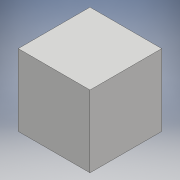
# Autodesk Inventor part: CalibrationCube
Saved by Autodesk Inventor 2017 (Build 210142000, 142)
## iProperties
Created: 2018-12-06
Part Number: CalibrationCube
Material: Generic
Document SubType Name: Modeling
Designer: Eric the Great
Density: 1 g/cm^3
Appearance: Default
Author: Eric the Great
Autodesk Inventor part; units mm, degrees
ref_plane "YZ Plane" through (0, 0, 0) normal (1, 0, 0) x (0, 1, 0)
ref_plane "XZ Plane" through (0, 0, 0) normal (0, 1, 0) x (-1, 0, 0)
ref_plane "XY Plane" through (0, 0, 0) normal (0, 0, 1) x (1, 0, 0)
sketch "Sketch1" plane through (0, 0, 0) normal (0, 1, 0) x (-1, 0, 0)
  line L0 (-28.325, 28.325) -> (28.325, 28.325)
  line L1 (28.325, 28.325) -> (28.325, -28.325)
  line L2 (28.325, -28.325) -> (-28.325, -28.325)
  line L3 (-28.325, -28.325) -> (-28.325, 28.325)
  line L4 (-28.325, 28.325) -> (28.325, -28.325) construction
  line L5 (28.325, 28.325) -> (-28.325, -28.325) construction
  point P0 (0, 0)
  dimension "d1" = 56.65
  constraints: 12 end point, 2 midpoint, 2 parallel, 2 perpendicular, 1 horizontal
  measures "d1" distance of L0.end L1.end
extrude "Extrusion1" add sketch "Sketch1" along normal blind 56.65
sketch "Sketch2" plane through (0, 56.65, 0) normal (0, 1, 0) x (1, 0, 0)
  line L0 (-16.1842, -24.3423) -> (-16.1842, 20.4869) construction
  line L1 (-16.1842, 20.4869) -> (-7.9053, 20.4869) construction
  line L2 (-7.9053, 20.4869) -> (-7.9053, -24.3423) construction
  line L3 (-7.9053, -24.3423) -> (-16.1842, -24.3423) construction
  line L4 (-0.0592, -21.5544) -> (-0.0592, 23.2747) construction
  line L5 (-0.0592, 23.2747) -> (5.9092, 23.2747) construction
  line L6 (5.9092, 23.2747) -> (5.9092, -21.5544) construction
  line L7 (5.9092, -21.5544) -> (-0.0592, -21.5544) construction
  line L8 (-8.6359, -18.0855) -> (-8.6359, -19.371)
  line L9 (-8.6359, -19.371) -> (-11.6211, -21.3753)
  line L10 (-11.6211, -21.3753) -> (-11.6211, -22.3927)
  line L11 (-11.6211, -22.3927) -> (-8.6359, -22.3927)
  line L12 (-8.6359, -22.3927) -> (-8.6359, -23.4345)
  line L13 (-8.6359, -23.4345) -> (-15.6359, -23.4345)
  line L14 (-15.6359, -23.4345) -> (-15.6359, -20.9793)
  spline S0 degree 2 poles (-15.6359, -20.9793) (-15.6359, -19.6634) (-15.1059, -18.5181) (-14.2652, -18.5181) knots 0 0 0 1 2 2 2
  line L15 (-14.2652, -18.5181) -> (-13.0589, -18.5181)
  spline S1 degree 2 poles (-13.0589, -18.5181) (-12.4131, -18.5181) (-11.7552, -19.5781) (-11.7552, -20.3336) knots 0 0 0 1 2 2 2
  line L16 (-11.7552, -20.3336) -> (-8.6359, -18.0855)
  line L17 (-13.1868, -19.5659) -> (-14.1555, -19.5659)
  spline S2 degree 2 poles (-14.1555, -19.5659) (-14.9414, -19.5659) (-14.9414, -20.9245) knots 0 0 0 1 1 1
  line L18 (-14.9414, -20.9245) -> (-14.9414, -22.3927)
  line L19 (-14.9414, -22.3927) -> (-12.3157, -22.3927)
  line L20 (-12.3157, -22.3927) -> (-12.3157, -21.022)
  spline S3 degree 2 poles (-12.3157, -21.022) (-12.3157, -20.2787) (-12.6812, -19.5659) (-13.1868, -19.5659) knots 0 0 0 1 2 2 2
  line L21 (-12.0963, -12.2857) -> (-10.2869, -12.2857)
  spline S4 degree 2 poles (-10.2869, -12.2857) (-9.7996, -12.2857) (-9.1294, -12.5233) (-8.7639, -12.8888) (-8.5689, -13.5712) (-8.5263, -14.1865) (-8.5263, -14.6921) knots 0 0 0 1 2 3 4 5 5 5
  spline S5 degree 2 poles (-8.5263, -14.6921) (-8.5263, -15.3379) (-8.6116, -16.0629) (-8.9466, -16.7818) (-9.6838, -17.0986) (-10.2869, -17.0986) knots 0 0 0 1 2 3 4 4 4
  line L22 (-10.2869, -17.0986) -> (-12.0963, -17.0986)
  spline S6 degree 2 poles (-12.0963, -17.0986) (-12.6142, -17.0986) (-13.327, -16.8488) (-13.7169, -16.4954) (-13.9179, -15.8009) (-13.9606, -15.21) (-13.9606, -14.1743) (-13.9179, -13.5833) (-13.7169, -12.8888) (-13.327, -12.5355) (-12.6142, -12.2857) (-12.0963, -12.2857) knots 0 0 0 1 2 3 4 5 6 7 8 9 10 10 10
  line L23 (-10.1468, -13.2787) -> (-12.2608, -13.2787)
  spline S7 degree 2 poles (-12.2608, -13.2787) (-12.9797, -13.2787) (-13.327, -13.8636) (-13.327, -15.5207) (-12.9797, -16.1055) (-12.2608, -16.1055) knots 0 0 0 1 2 3 4 4 4
  line L24 (-12.2608, -16.1055) -> (-10.1468, -16.1055)
  spline S8 degree 2 poles (-10.1468, -16.1055) (-9.7996, -16.1055) (-9.3914, -15.9532) (-9.2086, -15.5451) (-9.166, -15.1125) (-9.166, -14.2718) (-9.2086, -13.8392) (-9.3914, -13.431) (-9.7996, -13.2787) (-10.1468, -13.2787) knots 0 0 0 1 2 3 4 5 6 7 8 8 8
  line L25 (-12.4862, -6.0229) -> (-10.3418, -6.0229)
  spline S9 degree 2 poles (-10.3418, -6.0229) (-9.8666, -6.0229) (-9.1781, -6.3031) (-8.8004, -6.7235) (-8.5811, -7.418) (-8.5263, -8.0211) (-8.5263, -8.4537) knots 0 0 0 1 2 3 4 5 5 5
  spline S10 degree 2 poles (-8.5263, -8.4537) (-8.5263, -9.0142) (-8.6359, -9.7209) (-8.9832, -10.4337) (-9.7447, -10.7809) (-10.3418, -10.7809) knots 0 0 0 1 2 3 4 4 4
  line L26 (-10.3418, -10.7809) -> (-16.1842, -10.7809)
  line L27 (-16.1842, -10.7809) -> (-16.1842, -9.8122)
  line L28 (-16.1842, -9.8122) -> (-14.6185, -9.8122)
  spline S11 degree 2 poles (-14.6185, -9.8122) (-14.4175, -9.8122) (-13.5828, -9.8183) (-13.3818, -9.8183) knots 0 0 0 1 2 2 2
  spline S12 degree 2 poles (-13.3818, -9.8183) (-13.6316, -9.7757) (-13.9606, -8.9715) (-13.9606, -8.1795) knots 0 0 0 1 2 2 2
  spline S13 degree 2 poles (-13.9606, -8.1795) (-13.9606, -6.0229) (-12.4862, -6.0229) knots 0 0 0 1 1 1
  line L29 (-10.2016, -7.0159) -> (-12.2486, -7.0159)
  spline S14 degree 2 poles (-12.2486, -7.0159) (-12.9188, -7.0159) (-13.2721, -7.6434) (-13.2721, -8.4415) knots 0 0 0 1 2 2 2
  spline S15 degree 2 poles (-13.2721, -8.4415) (-13.2721, -9.2091) (-12.864, -9.8122) (-12.2486, -9.8122) knots 0 0 0 1 2 2 2
  line L30 (-12.2486, -9.8122) -> (-10.2016, -9.8122)
  spline S16 degree 2 poles (-10.2016, -9.8122) (-9.5437, -9.8122) (-9.166, -9.2152) (-9.166, -8.4293) knots 0 0 0 1 2 2 2
  spline S17 degree 2 poles (-9.166, -8.4293) (-9.166, -7.6312) (-9.5437, -7.0159) (-10.2016, -7.0159) knots 0 0 0 1 2 2 2
  line L31 (-12.0963, 0.0816) -> (-10.2869, 0.0816)
  spline S18 degree 2 poles (-10.2869, 0.0816) (-9.7996, 0.0816) (-9.1294, -0.156) (-8.7639, -0.5216) (-8.5689, -1.2039) (-8.5263, -1.8192) (-8.5263, -2.3249) knots 0 0 0 1 2 3 4 5 5 5
  spline S19 degree 2 poles (-8.5263, -2.3249) (-8.5263, -2.9706) (-8.6116, -3.6956) (-8.9466, -4.4145) (-9.6838, -4.7313) (-10.2869, -4.7313) knots 0 0 0 1 2 3 4 4 4
  line L32 (-10.2869, -4.7313) -> (-12.0963, -4.7313)
  spline S20 degree 2 poles (-12.0963, -4.7313) (-12.6142, -4.7313) (-13.327, -4.4815) (-13.7169, -4.1282) (-13.9179, -3.4337) (-13.9606, -2.8427) (-13.9606, -1.807) (-13.9179, -1.2161) (-13.7169, -0.5216) (-13.327, -0.1682) (-12.6142, 0.0816) (-12.0963, 0.0816) knots 0 0 0 1 2 3 4 5 6 7 8 9 10 10 10
  line L33 (-10.1468, -0.9115) -> (-12.2608, -0.9115)
  spline S21 degree 2 poles (-12.2608, -0.9115) (-12.9797, -0.9115) (-13.327, -1.4963) (-13.327, -3.1534) (-12.9797, -3.7383) (-12.2608, -3.7383) knots 0 0 0 1 2 3 4 4 4
  line L34 (-12.2608, -3.7383) -> (-10.1468, -3.7383)
  spline S22 degree 2 poles (-10.1468, -3.7383) (-9.7996, -3.7383) (-9.3914, -3.586) (-9.2086, -3.1778) (-9.166, -2.7452) (-9.166, -1.9045) (-9.2086, -1.4719) (-9.3914, -1.0638) (-9.7996, -0.9115) (-10.1468, -0.9115) knots 0 0 0 1 2 3 4 5 6 7 8 8 8
  spline S23 degree 2 poles (-8.6786, 5.3636) (-8.5263, 4.6508) (-8.5263, 3.6882) knots 0 0 0 1 1 1
  spline S24 degree 2 poles (-8.5263, 3.6882) (-8.5263, 3.213) (-8.5628, 2.6891) (-8.7456, 2.0067) (-9.0868, 1.6534) (-9.7447, 1.3914) (-10.2321, 1.3914) knots 0 0 0 1 2 3 4 5 5 5
  line L35 (-10.2321, 1.3914) -> (-12.1512, 1.3914)
  spline S25 degree 2 poles (-12.1512, 1.3914) (-12.5837, 1.3914) (-13.2051, 1.5559) (-13.595, 1.8971) (-13.8326, 2.2687) (-13.9301, 2.9023) (-13.9606, 3.3897) (-13.9606, 3.7979) knots 0 0 0 1 2 3 4 5 6 6 6
  spline S26 degree 2 poles (-13.9606, 3.7979) (-13.9606, 4.5411) (-13.8022, 5.2844) knots 0 0 0 1 1 1
  line L36 (-13.8022, 5.2844) -> (-13.0894, 5.2844)
  spline S27 degree 2 poles (-13.0894, 5.2844) (-13.3026, 4.4436) (-13.3026, 3.676) knots 0 0 0 1 1 1
  spline S28 degree 2 poles (-13.3026, 3.676) (-13.3026, 2.8718) (-12.9188, 2.3844) (-12.2913, 2.3844) knots 0 0 0 1 2 2 2
  line L37 (-12.2913, 2.3844) -> (-10.159, 2.3844)
  spline S29 degree 2 poles (-10.159, 2.3844) (-9.5863, 2.3844) (-9.2086, 2.9328) (-9.2086, 3.7857) knots 0 0 0 1 2 2 2
  spline S30 degree 2 poles (-9.2086, 3.7857) (-9.2086, 4.5533) (-9.4096, 5.3636) knots 0 0 0 1 1 1
  line L38 (-9.4096, 5.3636) -> (-8.6786, 5.3636)
  line L39 (-8.6359, 11.0842) -> (-8.6359, 10.1155)
  line L40 (-8.6359, 10.1155) -> (-9.2695, 10.1155)
  spline S31 degree 2 poles (-9.2695, 10.1155) (-8.5263, 9.9632) (-8.5263, 8.3975) knots 0 0 0 1 1 1
  spline S32 degree 2 poles (-8.5263, 8.3975) (-8.5263, 7.3679) (-9.2695, 6.5881) (-10.025, 6.5881) knots 0 0 0 1 2 2 2
  line L41 (-10.025, 6.5881) -> (-13.857, 6.5881)
  line L42 (-13.857, 6.5881) -> (-13.857, 7.5568)
  line L43 (-13.857, 7.5568) -> (-10.0798, 7.5568)
  spline S33 degree 2 poles (-10.0798, 7.5568) (-9.8848, 7.5568) (-9.629, 7.6238) (-9.3609, 7.8309) (-9.2208, 8.3122) (-9.2208, 8.6777) knots 0 0 0 1 2 3 4 4 4
  spline S34 degree 2 poles (-9.2208, 8.6777) (-9.2208, 9.488) (-9.5193, 10.1155) (-9.9214, 10.1155) knots 0 0 0 1 2 2 2
  line L44 (-9.9214, 10.1155) -> (-13.857, 10.1155)
  line L45 (-13.857, 10.1155) -> (-13.857, 11.0842)
  line L46 (-13.857, 11.0842) -> (-8.6359, 11.0842)
  line L47 (-12.4862, 17.5237) -> (-10.3418, 17.5237)
  spline S35 degree 2 poles (-10.3418, 17.5237) (-9.8666, 17.5237) (-9.1781, 17.2435) (-8.8004, 16.8231) (-8.5811, 16.1286) (-8.5263, 15.5254) (-8.5263, 15.0929) knots 0 0 0 1 2 3 4 5 5 5
  spline S36 degree 2 poles (-8.5263, 15.0929) (-8.5263, 14.5324) (-8.6359, 13.8257) (-8.9832, 13.1129) (-9.7447, 12.7657) (-10.3418, 12.7657) knots 0 0 0 1 2 3 4 4 4
  line L48 (-10.3418, 12.7657) -> (-16.1842, 12.7657)
  line L49 (-16.1842, 12.7657) -> (-16.1842, 13.7343)
  line L50 (-16.1842, 13.7343) -> (-14.6185, 13.7343)
  spline S37 degree 2 poles (-14.6185, 13.7343) (-14.4175, 13.7343) (-13.5828, 13.7282) (-13.3818, 13.7282) knots 0 0 0 1 2 2 2
  spline S38 degree 2 poles (-13.3818, 13.7282) (-13.6316, 13.7709) (-13.9606, 14.5751) (-13.9606, 15.367) knots 0 0 0 1 2 2 2
  spline S39 degree 2 poles (-13.9606, 15.367) (-13.9606, 17.5237) (-12.4862, 17.5237) knots 0 0 0 1 1 1
  line L51 (-10.2016, 16.5307) -> (-12.2486, 16.5307)
  spline S40 degree 2 poles (-12.2486, 16.5307) (-12.9188, 16.5307) (-13.2721, 15.9032) (-13.2721, 15.1051) knots 0 0 0 1 2 2 2
  spline S41 degree 2 poles (-13.2721, 15.1051) (-13.2721, 14.3375) (-12.864, 13.7343) (-12.2486, 13.7343) knots 0 0 0 1 2 2 2
  line L52 (-12.2486, 13.7343) -> (-10.2016, 13.7343)
  spline S42 degree 2 poles (-10.2016, 13.7343) (-9.5437, 13.7343) (-9.166, 14.3314) (-9.166, 15.1173) knots 0 0 0 1 2 2 2
  spline S43 degree 2 poles (-9.166, 15.1173) (-9.166, 15.9153) (-9.5437, 16.5307) (-10.2016, 16.5307) knots 0 0 0 1 2 2 2
  line L53 (-11.0302, 23.3053) -> (-11.0302, 19.7961)
  line L54 (-11.0302, 19.7961) -> (-10.2443, 19.7961)
  spline S44 degree 2 poles (-10.2443, 19.7961) (-9.6899, 19.7961) (-9.2269, 20.5759) (-9.2269, 21.3375) knots 0 0 0 1 2 2 2
  spline S45 degree 2 poles (-9.2269, 21.3375) (-9.2269, 22.0868) (-9.4888, 23.0981) knots 0 0 0 1 1 1
  line L55 (-9.4888, 23.0981) -> (-8.7456, 23.0981)
  spline S46 degree 2 poles (-8.7456, 23.0981) (-8.5263, 22.1294) (-8.5263, 21.2095) knots 0 0 0 1 1 1
  spline S47 degree 2 poles (-8.5263, 21.2095) (-8.5263, 18.8153) (-10.1224, 18.8153) knots 0 0 0 1 1 1
  line L56 (-10.1224, 18.8153) -> (-12.1816, 18.8153)
  spline S48 degree 2 poles (-12.1816, 18.8153) (-13.1442, 18.8153) (-13.9606, 19.918) (-13.9606, 21.1242) knots 0 0 0 1 2 2 2
  spline S49 degree 2 poles (-13.9606, 21.1242) (-13.9606, 22.2574) (-13.1747, 23.3053) (-12.1816, 23.3053) knots 0 0 0 1 2 2 2
  line L57 (-12.1816, 23.3053) -> (-11.0302, 23.3053)
  line L58 (-11.6638, 22.3305) -> (-12.4862, 22.3305)
  spline S50 degree 2 poles (-12.4862, 22.3305) (-12.9614, 22.3305) (-13.3148, 21.7517) (-13.3148, 21.0694) knots 0 0 0 1 2 2 2
  spline S51 degree 2 poles (-13.3148, 21.0694) (-13.3148, 20.4236) (-12.9736, 19.7961) (-12.4862, 19.7961) knots 0 0 0 1 2 2 2
  line L59 (-12.4862, 19.7961) -> (-11.6638, 19.7961)
  line L60 (-11.6638, 19.7961) -> (-11.6638, 22.3305)
  line L61 (2.054, 0.15) -> (3.2794, 0.15)
  spline S52 degree 2 poles (3.2794, 0.15) (3.5509, 0.15) (3.9443, -0.0102) (4.1601, -0.2504) (4.2855, -0.6472) (4.3168, -0.9919) (4.3168, -1.2391) knots 0 0 0 1 2 3 4 5 5 5
  spline S53 degree 2 poles (4.3168, -1.2391) (4.3168, -1.5593) (4.2541, -1.9632) (4.0557, -2.3705) (3.6205, -2.5689) (3.2794, -2.5689) knots 0 0 0 1 2 3 4 4 4
  line L62 (3.2794, -2.5689) -> (-0.0592, -2.5689)
  line L63 (-0.0592, -2.5689) -> (-0.0592, -2.0154)
  line L64 (-0.0592, -2.0154) -> (0.8355, -2.0154)
  spline S54 degree 2 poles (0.8355, -2.0154) (0.9504, -2.0154) (1.4273, -2.0189) (1.5422, -2.0189) knots 0 0 0 1 2 2 2
  spline S55 degree 2 poles (1.5422, -2.0189) (1.3995, -1.9945) (1.2115, -1.535) (1.2115, -1.0824) knots 0 0 0 1 2 2 2
  spline S56 degree 2 poles (1.2115, -1.0824) (1.2115, 0.15) (2.054, 0.15) knots 0 0 0 1 1 1
  line L65 (3.3594, -0.4175) -> (2.1897, -0.4175)
  spline S57 degree 2 poles (2.1897, -0.4175) (1.8068, -0.4175) (1.6049, -0.776) (1.6049, -1.2321) knots 0 0 0 1 2 2 2
  spline S58 degree 2 poles (1.6049, -1.2321) (1.6049, -1.6707) (1.8381, -2.0154) (2.1897, -2.0154) knots 0 0 0 1 2 2 2
  line L66 (2.1897, -2.0154) -> (3.3594, -2.0154)
  spline S59 degree 2 poles (3.3594, -2.0154) (3.7354, -2.0154) (3.9513, -1.6742) (3.9513, -1.2251) knots 0 0 0 1 2 2 2
  spline S60 degree 2 poles (3.9513, -1.2251) (3.9513, -0.7691) (3.7354, -0.4175) (3.3594, -0.4175) knots 0 0 0 1 2 2 2
  line L67 (1.2707, 3.318) -> (5.5352, 1.8175)
  line L68 (5.5352, 1.8175) -> (5.5352, 1.2396)
  line L69 (5.5352, 1.2396) -> (4.2959, 1.7096)
  line L70 (4.2959, 1.7096) -> (1.2707, 0.5573)
  line L71 (1.2707, 0.5573) -> (1.2707, 1.1596)
  line L72 (1.2707, 1.1596) -> (3.7041, 1.9916)
  line L73 (3.7041, 1.9916) -> (3.7041, 2.0055)
  line L74 (3.7041, 2.0055) -> (1.2707, 2.7575)
  line L75 (1.2707, 2.7575) -> (1.2707, 3.318)
  line L76 (10.6666, -11.8692) -> (10.6666, -12.6037)
  line L77 (10.6666, -12.6037) -> (8.9608, -13.7491)
  line L78 (8.9608, -13.7491) -> (8.9608, -14.3304)
  line L79 (8.9608, -14.3304) -> (10.6666, -14.3304)
  line L80 (10.6666, -14.3304) -> (10.6666, -14.9257)
  line L81 (10.6666, -14.9257) -> (6.6666, -14.9257)
  line L82 (6.6666, -14.9257) -> (6.6666, -13.5228)
  spline S61 degree 2 poles (6.6666, -13.5228) (6.6666, -12.7708) (6.9695, -12.1163) (7.4499, -12.1163) knots 0 0 0 1 2 2 2
  line L83 (7.4499, -12.1163) -> (8.1392, -12.1163)
  spline S62 degree 2 poles (8.1392, -12.1163) (8.5082, -12.1163) (8.8842, -12.7221) (8.8842, -13.1538) knots 0 0 0 1 2 2 2
  line L84 (8.8842, -13.1538) -> (10.6666, -11.8692)
  line L85 (8.0661, -12.7151) -> (7.5125, -12.7151)
  spline S63 degree 2 poles (7.5125, -12.7151) (7.0635, -12.7151) (7.0635, -13.4914) knots 0 0 0 1 1 1
  line L86 (7.0635, -13.4914) -> (7.0635, -14.3304)
  line L87 (7.0635, -14.3304) -> (8.5639, -14.3304)
  line L88 (8.5639, -14.3304) -> (8.5639, -13.5471)
  spline S64 degree 2 poles (8.5639, -13.5471) (8.5639, -13.1224) (8.355, -12.7151) (8.0661, -12.7151) knots 0 0 0 1 2 2 2
  line L89 (8.6892, -8.555) -> (9.7232, -8.555)
  spline S65 degree 2 poles (9.7232, -8.555) (10.0017, -8.555) (10.3846, -8.6907) (10.5935, -8.8996) (10.7049, -9.2895) (10.7292, -9.6411) (10.7292, -9.9301) knots 0 0 0 1 2 3 4 5 5 5
  spline S66 degree 2 poles (10.7292, -9.9301) (10.7292, -10.2991) (10.6805, -10.7134) (10.489, -11.1242) (10.0678, -11.3052) (9.7232, -11.3052) knots 0 0 0 1 2 3 4 4 4
  line L90 (9.7232, -11.3052) -> (8.6892, -11.3052)
  spline S67 degree 2 poles (8.6892, -11.3052) (8.3933, -11.3052) (7.986, -11.1625) (7.7632, -10.9605) (7.6483, -10.5637) (7.6239, -10.226) (7.6239, -9.6342) (7.6483, -9.2965) (7.7632, -8.8996) (7.986, -8.6977) (8.3933, -8.555) (8.6892, -8.555) knots 0 0 0 1 2 3 4 5 6 7 8 9 10 10 10
  line L91 (9.8032, -9.1224) -> (8.5952, -9.1224)
  spline S68 degree 2 poles (8.5952, -9.1224) (8.1844, -9.1224) (7.986, -9.4566) (7.986, -10.4035) (8.1844, -10.7377) (8.5952, -10.7377) knots 0 0 0 1 2 3 4 4 4
  line L92 (8.5952, -10.7377) -> (9.8032, -10.7377)
  spline S69 degree 2 poles (9.8032, -10.7377) (10.0017, -10.7377) (10.2349, -10.6507) (10.3393, -10.4175) (10.3637, -10.1703) (10.3637, -9.6899) (10.3393, -9.4427) (10.2349, -9.2095) (10.0017, -9.1224) (9.8032, -9.1224) knots 0 0 0 1 2 3 4 5 6 7 8 8 8
  line L93 (10.6666, -5.1259) -> (10.6666, -5.6794)
  line L94 (10.6666, -5.6794) -> (8.5082, -5.6794)
  spline S70 degree 2 poles (8.5082, -5.6794) (8.4003, -5.6794) (8.2506, -5.7177) (8.0974, -5.8326) (8.0173, -6.1111) (8.0173, -6.32) knots 0 0 0 1 2 3 4 4 4
  spline S71 degree 2 poles (8.0173, -6.32) (8.0173, -6.8074) (8.2262, -7.1416) (8.5082, -7.1416) knots 0 0 0 1 2 2 2
  line L95 (8.5082, -7.1416) -> (10.6666, -7.1416)
  line L96 (10.6666, -7.1416) -> (10.6666, -7.6951)
  line L97 (10.6666, -7.6951) -> (7.6831, -7.6951)
  line L98 (7.6831, -7.6951) -> (7.6831, -7.1416)
  line L99 (7.6831, -7.1416) -> (8.0487, -7.1416)
  spline S72 degree 2 poles (8.0487, -7.1416) (7.6239, -7.0545) (7.6239, -6.1599) knots 0 0 0 1 1 1
  spline S73 degree 2 poles (7.6239, -6.1599) (7.6239, -5.568) (8.0487, -5.1259) (8.4803, -5.1259) knots 0 0 0 1 2 2 2
  line L100 (8.4803, -5.1259) -> (10.6666, -5.1259)
  line L101 (8.4664, -1.4462) -> (9.6918, -1.4462)
  spline S74 degree 2 poles (9.6918, -1.4462) (9.9634, -1.4462) (10.3568, -1.6063) (10.5726, -1.8465) (10.6979, -2.2434) (10.7292, -2.5881) (10.7292, -2.8352) knots 0 0 0 1 2 3 4 5 5 5
  spline S75 degree 2 poles (10.7292, -2.8352) (10.7292, -3.1555) (10.6666, -3.5593) (10.4682, -3.9666) (10.033, -4.1651) (9.6918, -4.1651) knots 0 0 0 1 2 3 4 4 4
  line L102 (9.6918, -4.1651) -> (6.3533, -4.1651)
  line L103 (6.3533, -4.1651) -> (6.3533, -3.6115)
  line L104 (6.3533, -3.6115) -> (7.248, -3.6115)
  spline S76 degree 2 poles (7.248, -3.6115) (7.3628, -3.6115) (7.8398, -3.615) (7.9547, -3.615) knots 0 0 0 1 2 2 2
  spline S77 degree 2 poles (7.9547, -3.615) (7.8119, -3.5907) (7.6239, -3.1311) (7.6239, -2.6786) knots 0 0 0 1 2 2 2
  spline S78 degree 2 poles (7.6239, -2.6786) (7.6239, -1.4462) (8.4664, -1.4462) knots 0 0 0 1 1 1
  line L105 (9.7719, -2.0136) -> (8.6022, -2.0136)
  spline S79 degree 2 poles (8.6022, -2.0136) (8.2192, -2.0136) (8.0173, -2.3722) (8.0173, -2.8283) knots 0 0 0 1 2 2 2
  spline S80 degree 2 poles (8.0173, -2.8283) (8.0173, -3.2669) (8.2506, -3.6115) (8.6022, -3.6115) knots 0 0 0 1 2 2 2
  line L106 (8.6022, -3.6115) -> (9.7719, -3.6115)
  spline S81 degree 2 poles (9.7719, -3.6115) (10.1479, -3.6115) (10.3637, -3.2704) (10.3637, -2.8213) knots 0 0 0 1 2 2 2
  spline S82 degree 2 poles (10.3637, -2.8213) (10.3637, -2.3652) (10.1479, -2.0136) (9.7719, -2.0136) knots 0 0 0 1 2 2 2
  line L107 (9.2984, 1.8576) -> (9.2984, -0.1477)
  line L108 (9.2984, -0.1477) -> (9.7475, -0.1477)
  spline S83 degree 2 poles (9.7475, -0.1477) (10.0643, -0.1477) (10.3289, 0.2979) (10.3289, 0.7331) knots 0 0 0 1 2 2 2
  spline S84 degree 2 poles (10.3289, 0.7331) (10.3289, 1.1613) (10.1792, 1.7392) knots 0 0 0 1 1 1
  line L109 (10.1792, 1.7392) -> (10.6039, 1.7392)
  spline S85 degree 2 poles (10.6039, 1.7392) (10.7292, 1.1857) (10.7292, 0.66) knots 0 0 0 1 1 1
  spline S86 degree 2 poles (10.7292, 0.66) (10.7292, -0.7082) (9.8172, -0.7082) knots 0 0 0 1 1 1
  line L110 (9.8172, -0.7082) -> (8.6405, -0.7082)
  spline S87 degree 2 poles (8.6405, -0.7082) (8.0904, -0.7082) (7.6239, -0.078) (7.6239, 0.6113) knots 0 0 0 1 2 2 2
  spline S88 degree 2 poles (7.6239, 0.6113) (7.6239, 1.2588) (8.073, 1.8576) (8.6405, 1.8576) knots 0 0 0 1 2 2 2
  line L111 (8.6405, 1.8576) -> (9.2984, 1.8576)
  line L112 (8.9364, 1.3005) -> (8.4664, 1.3005)
  spline S89 degree 2 poles (8.4664, 1.3005) (8.1949, 1.3005) (7.993, 0.9698) (7.993, 0.5799) knots 0 0 0 1 2 2 2
  spline S90 degree 2 poles (7.993, 0.5799) (7.993, 0.2109) (8.1879, -0.1477) (8.4664, -0.1477) knots 0 0 0 1 2 2 2
  line L113 (8.4664, -0.1477) -> (8.9364, -0.1477)
  line L114 (8.9364, -0.1477) -> (8.9364, 1.3005)
  line L115 (8.0974, 4.3084) -> (8.0974, 4.002)
  spline S91 degree 2 poles (8.0974, 4.002) (8.0974, 3.6191) (8.2958, 3.2536) (8.5639, 3.2536) knots 0 0 0 1 2 2 2
  line L116 (8.5639, 3.2536) -> (10.6666, 3.2536)
  line L117 (10.6666, 3.2536) -> (10.6666, 2.7)
  line L118 (10.6666, 2.7) -> (7.6831, 2.7)
  line L119 (7.6831, 2.7) -> (7.6831, 3.2257)
  line L120 (7.6831, 3.2257) -> (8.1705, 3.2257)
  spline S92 degree 2 poles (8.1705, 3.2257) (7.9547, 3.2257) (7.6239, 3.7618) (7.6239, 4.0368) knots 0 0 0 1 2 2 2
  line L121 (7.6239, 4.0368) -> (7.6239, 4.3084)
  line L122 (7.6239, 4.3084) -> (8.0974, 4.3084)
  line L123 (7.6831, 7.4067) -> (10.9486, 7.4067)
  spline S93 degree 2 poles (10.9486, 7.4067) (11.5856, 7.4067) (12.0208, 6.7) (12.0208, 5.9898) knots 0 0 0 1 2 2 2
  spline S94 degree 2 poles (12.0208, 5.9898) (12.0208, 5.3562) (11.9547, 4.9594) knots 0 0 0 1 1 1
  line L124 (11.9547, 4.9594) -> (11.5613, 4.9594)
  spline S95 degree 2 poles (11.5613, 4.9594) (11.6448, 5.6696) (11.6448, 6.0386) knots 0 0 0 1 1 1
  spline S96 degree 2 poles (11.6448, 6.0386) (11.6448, 6.4633) (11.3768, 6.8532) (11.06, 6.8532) knots 0 0 0 1 2 2 2
  line L125 (11.06, 6.8532) -> (10.3463, 6.8532)
  spline S97 degree 2 poles (10.3463, 6.8532) (10.5552, 6.8393) (10.7292, 6.2927) (10.7292, 5.9411) knots 0 0 0 1 2 2 2
  spline S98 degree 2 poles (10.7292, 5.9411) (10.7292, 5.2518) (10.3219, 4.7505) (9.8241, 4.7505) knots 0 0 0 1 2 2 2
  line L126 (9.8241, 4.7505) -> (8.6091, 4.7505)
  spline S99 degree 2 poles (8.6091, 4.7505) (8.08, 4.7505) (7.6239, 5.3249) (7.6239, 5.9759) knots 0 0 0 1 2 2 2
  spline S100 degree 2 poles (7.6239, 5.9759) (7.6239, 6.7522) (7.9756, 6.888) knots 0 0 0 1 1 1
  line L127 (7.9756, 6.888) -> (7.6831, 6.888)
  line L128 (7.6831, 6.888) -> (7.6831, 7.4067)
  line L129 (9.8589, 6.8532) -> (8.5082, 6.8532)
  spline S101 degree 2 poles (8.5082, 6.8532) (8.2192, 6.8532) (8.0034, 6.5399) (8.0034, 6.0455) knots 0 0 0 1 2 2 2
  spline S102 degree 2 poles (8.0034, 6.0455) (8.0034, 5.5825) (8.2158, 5.3005) (8.5082, 5.3005) knots 0 0 0 1 2 2 2
  line L130 (8.5082, 5.3005) -> (9.8589, 5.3005)
  spline S103 degree 2 poles (9.8589, 5.3005) (10.1688, 5.3005) (10.3568, 5.5999) (10.3568, 6.056) knots 0 0 0 1 2 2 2
  spline S104 degree 2 poles (10.3568, 6.056) (10.3568, 6.4772) (10.1548, 6.8532) (9.8589, 6.8532) knots 0 0 0 1 2 2 2
  line L131 (7.6831, 10.6861) -> (11.9477, 9.1857)
  line L132 (11.9477, 9.1857) -> (11.9477, 8.6078)
  line L133 (11.9477, 8.6078) -> (10.7084, 9.0777)
  line L134 (10.7084, 9.0777) -> (7.6831, 7.9254)
  line L135 (7.6831, 7.9254) -> (7.6831, 8.5277)
  line L136 (7.6831, 8.5277) -> (10.1165, 9.3597)
  line L137 (10.1165, 9.3597) -> (10.1165, 9.3737)
  line L138 (10.1165, 9.3737) -> (7.6831, 10.1256)
  line L139 (7.6831, 10.1256) -> (7.6831, 10.6861)
  line L140 (7.4568, 15.3719) -> (8.2889, 15.3719)
  spline S105 degree 2 poles (8.2889, 15.3719) (8.8006, 15.3719) (9.2253, 14.5782) (9.2253, 13.8506) knots 0 0 0 1 2 2 2
  line L141 (9.2253, 13.8506) -> (9.2253, 13.2518)
  line L142 (9.2253, 13.2518) -> (10.6666, 13.2518)
  line L143 (10.6666, 13.2518) -> (10.6666, 12.6565)
  line L144 (10.6666, 12.6565) -> (6.6666, 12.6565)
  line L145 (6.6666, 12.6565) -> (6.6666, 13.962)
  spline S106 degree 2 poles (6.6666, 13.962) (6.6666, 14.2092) (6.691, 14.5643) (6.785, 14.9646) (6.9521, 15.2048) (7.248, 15.3719) (7.4568, 15.3719) knots 0 0 0 1 2 3 4 5 5 5
  line L146 (8.2575, 14.7871) -> (7.5299, 14.7871)
  spline S107 degree 2 poles (7.5299, 14.7871) (7.3628, 14.7871) (7.147, 14.6165) (7.0635, 14.2962) (7.0426, 14.0804) (7.0426, 13.9202) knots 0 0 0 1 2 3 4 4 4
  line L147 (7.0426, 13.9202) -> (7.0426, 13.2483)
  line L148 (7.0426, 13.2483) -> (8.8494, 13.2483)
  line L149 (8.8494, 13.2483) -> (8.8494, 13.9307)
  spline S108 degree 2 poles (8.8494, 13.9307) (8.8494, 14.2892) (8.5848, 14.7871) (8.2575, 14.7871) knots 0 0 0 1 2 2 2
  line L150 (10.6666, 16.6844) -> (10.6666, 16.1308)
  line L151 (10.6666, 16.1308) -> (7.6831, 16.1308)
  line L152 (7.6831, 16.1308) -> (7.6831, 16.6844)
  line L153 (7.6831, 16.6844) -> (10.6666, 16.6844)
  line L154 (7.1853, 16.6844) -> (7.1853, 16.1308)
  line L155 (7.1853, 16.1308) -> (6.6074, 16.1308)
  line L156 (6.6074, 16.1308) -> (6.6074, 16.6844)
  line L157 (6.6074, 16.6844) -> (7.1853, 16.6844)
  point P0 (0, 0)
  constraints: 4 other
extrude "Extrusion2" cut sketch "Sketch2" against normal blind 2
body "Solid1"
